Autodesk Fusion 360 part; units mm, degrees
(part 2 of 2)
  spline S375 degree 3 poles (1.9158, -4.1555) (1.6856, -3.9558) (1.3163, -3.6912) (1.1005, -3.5598) knots 0 0 0 0 1 1 1 1
  spline S376 degree 3 poles (1.1005, -3.5598) (0.8754, -3.4317) (0.4108, -3.1073) (0.0566, -2.8267) knots 0 0 0 0 1 1 1 1
  spline S377 degree 3 poles (0.0566, -2.8267) (-0.2941, -2.5554) (-0.6989, -2.2512) (-0.8388, -2.1551) knots 0 0 0 0 1 1 1 1
  spline S378 degree 3 poles (-0.8388, -2.1551) (-0.9788, -2.059) (-1.3388, -1.7911) (-1.6449, -1.556) knots 0 0 0 0 1 1 1 1
  spline S379 degree 3 poles (-1.6449, -1.556) (-1.9417, -1.3175) (-2.3043, -1.0714) (-2.4341, -1.0032) knots 0 0 0 0 1 1 1 1
  spline S380 degree 3 poles (-2.4341, -1.0032) (-2.5639, -0.9349) (-2.7739, -0.7909) (-2.9046, -0.6914) knots 0 0 0 0 1 1 1 1
  spline S381 degree 3 poles (-2.9046, -0.6914) (-3.4695, -0.2355) (-3.9222, -0.4633) (-3.5882, -1.0347) knots 0 0 0 0 1 1 1 1
  spline S382 degree 3 poles (-3.5882, -1.0347) (-3.4574, -1.2496) (-3.4321, -1.3769) (-3.4978, -1.4849) knots 0 0 0 0 1 1 1 1
  spline S383 degree 3 poles (-3.4978, -1.4849) (-3.6891, -1.796) (-4.0336, -2.8979) (-4.0486, -3.2604) knots 0 0 0 0 1 1 1 1
  spline S384 degree 3 poles (-4.0486, -3.2604) (-4.0922, -4.1792) (-3.8414, -5.705) (-3.4803, -6.6971) knots 0 0 0 0 1 1 1 1
  spline S385 degree 3 poles (-3.4803, -6.6971) (-3.1361, -7.6428) (-3.1099, -7.6858) (-2.4943, -8.2808) knots 0 0 0 0 1 1 1 1
  spline S386 degree 3 poles (-2.4943, -8.2808) (-1.8788, -8.8758) (-1.453, -9.1513) (-0.5011, -9.6029) knots 0 0 0 0 1 1 1 1
  spline S387 degree 3 poles (-0.5011, -9.6029) (-0.0425, -9.8244) (1.2112, -10.1242) (1.3873, -10.06) knots 0 0 0 0 1 1 1 1
  spline S388 degree 3 poles (1.3873, -10.06) (1.4337, -10.0432) (1.765, -10.0591) (2.125, -10.0961) knots 0 0 0 0 1 1 1 1
  spline S389 degree 3 poles (2.125, -10.0961) (3.0076, -10.1843) (4.5443, -9.877) (5.7007, -9.3616) knots 0 0 0 0 1 1 1 1
  line L40 (5.7007, -9.3616) -> (6.5613, -8.9854)
  line L41 (6.5613, -8.9854) -> (6.9205, -9.2222)
  spline S390 degree 3 poles (6.9205, -9.2222) (7.1237, -9.3477) (7.3025, -9.4926) (7.3227, -9.5483) knots 0 0 0 0 1 1 1 1
  spline S391 degree 3 poles (7.3227, -9.5483) (7.3396, -9.5946) (7.4922, -9.6966) (7.6659, -9.7699) knots 0 0 0 0 1 1 1 1
  spline S392 degree 3 poles (7.6659, -9.7699) (7.9247, -9.8752) (8.0183, -9.8726) (8.1118, -9.7546) knots 0 0 0 0 1 1 1 1
  spline S393 degree 3 poles (8.1118, -9.7546) (8.2534, -9.5666) (8.2272, -9.2926) (8.0704, -9.2657) knots 0 0 0 0 1 1 1 1
  spline S394 degree 3 poles (5.741, -8.549) (5.6676, -8.6071) (5.0489, -8.8113) (4.3485, -8.9928) knots 0 0 0 0 1 1 1 1
  spline S395 degree 3 poles (4.3485, -8.9928) (3.0596, -9.3464) (2.0565, -9.4175) (0.8476, -9.2695) knots 0 0 0 0 1 1 1 1
  spline S396 degree 3 poles (0.8476, -9.2695) (0.0678, -9.1753) (-1.0477, -8.5628) (-1.8774, -7.7832) knots 0 0 0 0 1 1 1 1
  spline S397 degree 3 poles (-1.8774, -7.7832) (-2.2586, -7.4284) (-2.3859, -7.2228) (-2.7267, -6.4018) knots 0 0 0 0 1 1 1 1
  spline S398 degree 3 poles (-2.7267, -6.4018) (-3.0481, -5.6053) (-3.1283, -5.2985) (-3.1774, -4.6443) knots 0 0 0 0 1 1 1 1
  spline S399 degree 3 poles (-3.1774, -4.6443) (-3.2756, -3.336) (-3.0585, -1.913) (-2.734, -1.7948) knots 0 0 0 0 1 1 1 1
  spline S400 degree 3 poles (-2.734, -1.7948) (-2.6876, -1.778) (-2.5477, -1.874) (-2.4473, -2.0055) knots 0 0 0 0 1 1 1 1
  spline S401 degree 3 poles (-2.4473, -2.0055) (-2.3343, -2.1429) (-2.207, -2.2331) (-2.1606, -2.2162) knots 0 0 0 0 1 1 1 1
  spline S402 degree 3 poles (-2.1606, -2.2162) (-2.1143, -2.1993) (-1.981, -2.2768) (-1.8714, -2.4049) knots 0 0 0 0 1 1 1 1
  spline S403 degree 3 poles (-1.8714, -2.4049) (-1.7559, -2.5204) (-1.5232, -2.6982) (-1.3613, -2.7968) knots 0 0 0 0 1 1 1 1
  spline S404 degree 3 poles (-1.3613, -2.7968) (-1.1868, -2.9012) (-1.0367, -3.0251) (-1.0198, -3.0715) knots 0 0 0 0 1 1 1 1
  spline S405 degree 3 poles (-1.0198, -3.0715) (-0.9995, -3.1271) (-0.841, -3.2164) (-0.6707, -3.2804) knots 0 0 0 0 1 1 1 1
  line L42 (-0.6707, -3.2804) -> (-0.3647, -3.4001)
  line L43 (-0.3647, -3.4001) -> (-0.8376, -3.5722)
  spline S406 degree 3 poles (-0.8376, -3.5722) (-1.3475, -3.7578) (-1.4461, -3.9197) (-1.2437, -4.245) knots 0 0 0 0 1 1 1 1
  spline S407 degree 3 poles (-1.2437, -4.245) (-1.1062, -4.4785) (-0.6307, -4.5154) (0.2358, -4.3575) knots 0 0 0 0 1 1 1 1
  spline S408 degree 3 poles (0.2358, -4.3575) (0.7449, -4.2562) (0.7702, -4.268) (1.6868, -5.0264) knots 0 0 0 0 1 1 1 1
  spline S409 degree 3 poles (1.6868, -5.0264) (1.8976, -5.2017) (2.4237, -5.6087) (2.8698, -5.9399) knots 0 0 0 0 1 1 1 1
  spline S410 degree 3 poles (2.8698, -5.9399) (3.3192, -6.2803) (3.9094, -6.748) (4.1877, -6.9932) knots 0 0 0 0 1 1 1 1
  spline S411 degree 3 poles (4.1877, -6.9932) (4.466, -7.2385) (4.7788, -7.4921) (4.896, -7.5545) knots 0 0 0 0 1 1 1 1
  spline S412 degree 3 poles (4.896, -7.5545) (5.197, -7.7179) (5.7526, -8.1772) (5.8159, -8.3222) knots 0 0 0 0 1 1 1 1
  spline S413 degree 3 poles (5.8159, -8.3222) (5.8488, -8.3837) (5.8109, -8.4815) (5.741, -8.549) knots 0 0 0 0 1 1 1 1
  spline S414 degree 3 poles (-3.274, 16.9406) (-3.4561, 17.0948) (-3.6786, 17.0138) (-4.2602, 16.5921) knots 0 0 0 0 1 1 1 1
  spline S415 degree 3 poles (-4.2602, 16.5921) (-4.6917, 16.2775) (-4.7473, 16.2573) (-5.5009, 16.193) knots 0 0 0 0 1 1 1 1
  spline S416 degree 3 poles (-5.5009, 16.193) (-6.7435, 16.0873) (-8.9021, 15.2386) (-10.4235, 14.2543) knots 0 0 0 0 1 1 1 1
  spline S417 degree 3 poles (-10.4235, 14.2543) (-10.8128, 13.9971) (-11.605, 13.2888) (-12.2025, 12.6513) knots 0 0 0 0 1 1 1 1
  spline S418 degree 3 poles (-12.2025, 12.6513) (-13.352, 11.4244) (-15.0798, 7.4879) (-15.2033, 5.8365) knots 0 0 0 0 1 1 1 1
  spline S419 degree 3 poles (-15.2033, 5.8365) (-15.2159, 5.6114) (-15.2756, 5.2851) (-15.3236, 5.0997) knots 0 0 0 0 1 1 1 1
  spline S420 degree 3 poles (-15.3236, 5.0997) (-15.4323, 4.7346) (-15.4883, 3.1287) (-15.4347, 1.5102) knots 0 0 0 0 1 1 1 1
  spline S421 degree 3 poles (-15.4347, 1.5102) (-15.3878, -0.3208) (-14.9842, -2.295) (-14.2595, -4.2573) knots 0 0 0 0 1 1 1 1
  spline S422 degree 3 poles (-14.2595, -4.2573) (-13.8174, -5.4719) (-13.6622, -5.7829) (-13.0601, -6.6873) knots 0 0 0 0 1 1 1 1
  spline S423 degree 3 poles (-13.0601, -6.6873) (-12.5718, -7.4231) (-12.2201, -7.8411) (-11.8592, -8.1402) knots 0 0 0 0 1 1 1 1
  spline S424 degree 3 poles (-11.8592, -8.1402) (-11.5692, -8.3602) (-11.1374, -8.7385) (-10.8971, -8.9661) knots 0 0 0 0 1 1 1 1
  spline S425 degree 3 poles (-10.8971, -8.9661) (-10.4359, -9.3967) (-9.5489, -9.9874) (-8.7513, -10.3901) knots 0 0 0 0 1 1 1 1
  spline S426 degree 3 poles (-8.7513, -10.3901) (-7.9537, -10.7928) (-4.9869, -11.6451) (-4.718, -11.5472) knots 0 0 0 0 1 1 1 1
  spline S427 degree 3 poles (-4.718, -11.5472) (-4.4121, -11.4358) (-3.9341, -11.5664) (-2.8785, -12.0432) knots 0 0 0 0 1 1 1 1
  spline S428 degree 3 poles (-2.8785, -12.0432) (-1.7057, -12.5824) (-1.3795, -12.6421) (-1.3324, -12.31) knots 0 0 0 0 1 1 1 1
  spline S429 degree 3 poles (-1.3324, -12.31) (-1.3054, -12.1531) (-1.4429, -12.0352) (-2.0415, -11.7175) knots 0 0 0 0 1 1 1 1
  spline S430 degree 3 poles (-2.0415, -11.7175) (-2.447, -11.4976) (-2.8113, -11.3047) (-2.8585, -11.2904) knots 0 0 0 0 1 1 1 1
  spline S431 degree 3 poles (-2.8585, -11.2904) (-3.2075, -11.1969) (-4.9717, -9.1194) (-5.6253, -8.0448) knots 0 0 0 0 1 1 1 1
  spline S432 degree 3 poles (-5.6253, -8.0448) (-6.3675, -6.8134) (-6.6982, -6.0203) (-7.1606, -4.4035) knots 0 0 0 0 1 1 1 1
  spline S433 degree 3 poles (-7.1606, -4.4035) (-7.807, -2.1083) (-8.1042, -0.7149) (-8.1424, 0.2267) knots 0 0 0 0 1 1 1 1
  spline S434 degree 3 poles (-8.1424, 0.2267) (-8.1712, 0.7098) (-8.2212, 1.5106) (-8.266, 2.0088) knots 0 0 0 0 1 1 1 1
  spline S435 degree 3 poles (-8.266, 2.0088) (-8.4807, 4.1567) (-8.2895, 7.5549) (-7.8887, 8.8768) knots 0 0 0 0 1 1 1 1
  spline S436 degree 3 poles (-7.8887, 8.8768) (-7.7851, 9.198) (-7.6731, 9.6693) (-7.6361, 9.9137) knots 0 0 0 0 1 1 1 1
  spline S437 degree 3 poles (-7.6361, 9.9137) (-7.5376, 10.5376) (-7.3708, 10.9448) (-6.8249, 11.9835) knots 0 0 0 0 1 1 1 1
  spline S438 degree 3 poles (-6.8249, 11.9835) (-6.5637, 12.4776) (-6.2343, 13.1015) (-6.0919, 13.3739) knots 0 0 0 0 1 1 1 1
  spline S439 degree 3 poles (-6.0919, 13.3739) (-5.9529, 13.6555) (-5.8063, 13.8873) (-5.7784, 13.8974) knots 0 0 0 0 1 1 1 1
  spline S440 degree 3 poles (-5.7784, 13.8974) (-5.7414, 13.9109) (-5.545, 14.1504) (-5.3343, 14.4371) knots 0 0 0 0 1 1 1 1
  spline S441 degree 3 poles (-5.3343, 14.4371) (-4.8709, 15.0678) (-4.0425, 15.9363) (-3.5713, 16.2863) knots 0 0 0 0 1 1 1 1
  spline S442 degree 3 poles (-3.5713, 16.2863) (-3.1491, 16.5975) (-3.0724, 16.7619) (-3.274, 16.9406) knots 0 0 0 0 1 1 1 1
  spline S443 degree 3 poles (-6.1294, 14.8617) (-6.4572, 14.5219) (-7.5618, 12.5658) (-7.6477, 12.1671) knots 0 0 0 0 1 1 1 1
  spline S444 degree 3 poles (-7.6477, 12.1671) (-7.7504, 11.6992) (-7.7007, 11.7068) (-9.8958, 11.6218) knots 0 0 0 0 1 1 1 1
  spline S445 degree 3 poles (-9.8958, 11.6218) (-10.2574, 11.6057) (-10.8981, 11.5195) (-12.085, 11.3186) knots 0 0 0 0 1 1 1 1
  spline S446 degree 3 poles (-12.085, 11.3186) (-12.2713, 11.2822) (-12.1381, 11.4357) (-10.5706, 13.0143) knots 0 0 0 0 1 1 1 1
  spline S447 degree 3 poles (-10.5706, 13.0143) (-10.1181, 13.473) (-8.5225, 14.3687) (-7.0997, 14.9601) knots 0 0 0 0 1 1 1 1
  spline S448 degree 3 poles (-7.0997, 14.9601) (-5.8312, 15.4848) (-5.3254, 15.5954) (-5.7005, 15.2699) knots 0 0 0 0 1 1 1 1
  spline S449 degree 3 poles (-5.7005, 15.2699) (-5.8134, 15.1763) (-5.9988, 14.9933) (-6.1294, 14.8617) knots 0 0 0 0 1 1 1 1
  spline S450 degree 3 poles (-8.2095, 10.6815) (-8.2491, 10.6461) (-8.3553, 10.303) (-8.4538, 9.9101) knots 0 0 0 0 1 1 1 1
  spline S451 degree 3 poles (-8.4538, 9.9101) (-8.5523, 9.5173) (-8.6643, 9.1615) (-8.7064, 9.1042) knots 0 0 0 0 1 1 1 1
  spline S452 degree 3 poles (-8.7064, 9.1042) (-8.8151, 8.9701) (-9.0078, 7.7974) (-9.0085, 7.2512) knots 0 0 0 0 1 1 1 1
  spline S453 degree 3 poles (-9.0085, 7.2512) (-9.0193, 6.5017) (-9.1398, 6.3424) (-9.7307, 6.2638) knots 0 0 0 0 1 1 1 1
  spline S454 degree 3 poles (-9.7307, 6.2638) (-10.0013, 6.2283) (-10.3005, 6.2139) (-10.3882, 6.224) knots 0 0 0 0 1 1 1 1
  spline S455 degree 3 poles (-10.3882, 6.224) (-10.7642, 6.2761) (-12.8463, 6.0538) (-13.8494, 5.8672) knots 0 0 0 0 1 1 1 1
  spline S456 degree 3 poles (-13.8494, 5.8672) (-14.3181, 5.7701) (-14.4142, 5.8612) (-14.2879, 6.2641) knots 0 0 0 0 1 1 1 1
  spline S457 degree 3 poles (-14.2879, 6.2641) (-13.8635, 7.6367) (-13.6756, 8.188) (-13.5156, 8.6138) knots 0 0 0 0 1 1 1 1
  spline S458 degree 3 poles (-13.5156, 8.6138) (-13.4137, 8.8819) (-13.3362, 9.1306) (-13.3497, 9.1677) knots 0 0 0 0 1 1 1 1
  spline S459 degree 3 poles (-13.3497, 9.1677) (-13.3598, 9.1955) (-13.2208, 9.4771) (-13.0354, 9.7756) knots 0 0 0 0 1 1 1 1
  spline S460 degree 3 poles (-13.0354, 9.7756) (-12.7456, 10.2486) (-12.6267, 10.3548) (-12.2651, 10.4865) knots 0 0 0 0 1 1 1 1
  spline S461 degree 3 poles (-12.2651, 10.4865) (-11.8108, 10.6518) (-11.2696, 10.7228) (-10.6542, 10.7053) knots 0 0 0 0 1 1 1 1
  spline S462 degree 3 poles (-10.6542, 10.7053) (-10.4544, 10.7045) (-9.8155, 10.7376) (-9.2397, 10.8001) knots 0 0 0 0 1 1 1 1
  spline S463 degree 3 poles (-9.2397, 10.8001) (-8.3023, 10.8788) (-8.03, 10.8519) (-8.2095, 10.6815) knots 0 0 0 0 1 1 1 1
  spline S464 degree 3 poles (-9.1436, 4.997) (-9.2344, 4.3234) (-9.0243, 0.6303) (-8.8292, -0.5692) knots 0 0 0 0 1 1 1 1
  spline S465 degree 3 poles (-8.8292, -0.5692) (-8.7017, -1.3523) (-8.7118, -1.44) (-8.9014, -1.4671) knots 0 0 0 0 1 1 1 1
  spline S466 degree 3 poles (-8.9014, -1.4671) (-9.0102, -1.4856) (-9.4325, -1.5658) (-9.8329, -1.6486) knots 0 0 0 0 1 1 1 1
  spline S467 degree 3 poles (-9.8329, -1.6486) (-10.2333, -1.7313) (-10.9734, -1.8327) (-11.4809, -1.8809) knots 0 0 0 0 1 1 1 1
  spline S468 degree 3 poles (-11.4809, -1.8809) (-11.9791, -1.9257) (-12.7099, -2.0237) (-13.101, -2.1031) knots 0 0 0 0 1 1 1 1
  spline S469 degree 3 poles (-13.101, -2.1031) (-13.4829, -2.1791) (-13.8909, -2.212) (-14.0106, -2.1716) knots 0 0 0 0 1 1 1 1
  spline S470 degree 3 poles (-14.0106, -2.1716) (-14.2087, -2.1177) (-14.2222, -2.0806) (-14.2899, -1.3177) knots 0 0 0 0 1 1 1 1
  spline S471 degree 3 poles (-14.2899, -1.3177) (-14.3271, -0.8693) (-14.4015, -0.3188) (-14.4487, -0.0735) knots 0 0 0 0 1 1 1 1
  spline S472 degree 3 poles (-14.4487, -0.0735) (-14.6438, 0.895) (-14.7224, 4.573) (-14.5581, 4.9583) knots 0 0 0 0 1 1 1 1
  spline S473 degree 3 poles (-14.5581, 4.9583) (-14.511, 5.0594) (-12.1186, 5.3527) (-10.4858, 5.4535) knots 0 0 0 0 1 1 1 1
  spline S474 degree 3 poles (-10.4858, 5.4535) (-9.9311, 5.4873) (-9.4143, 5.5389) (-9.3494, 5.5625) knots 0 0 0 0 1 1 1 1
  spline S475 degree 3 poles (-9.3494, 5.5625) (-9.1825, 5.6233) (-9.0881, 5.3637) (-9.1436, 4.997) knots 0 0 0 0 1 1 1 1
  spline S476 degree 3 poles (-4.8203, -10.7759) (-5.1811, -10.7077) (-7.1202, -10.1114) (-8.0872, -9.7914) knots 0 0 0 0 1 1 1 1
  spline S477 degree 3 poles (-8.0872, -9.7914) (-8.292, -9.719) (-8.7321, -9.4906) (-9.0534, -9.2715) knots 0 0 0 0 1 1 1 1
  spline S478 degree 3 poles (-9.0534, -9.2715) (-9.3839, -9.0558) (-9.8282, -8.7871) (-10.0432, -8.6868) knots 0 0 0 0 1 1 1 1
  spline S479 degree 3 poles (-10.0432, -8.6868) (-10.2523, -8.5739) (-10.3957, -8.4686) (-10.34, -8.4483) knots 0 0 0 0 1 1 1 1
  spline S480 degree 3 poles (-10.34, -8.4483) (-10.2937, -8.4314) (-9.7213, -8.3596) (-9.0646, -8.2886) knots 0 0 0 0 1 1 1 1
  spline S481 degree 3 poles (-9.0646, -8.2886) (-8.4046, -8.2269) (-7.6274, -8.112) (-7.3357, -8.0479) knots 0 0 0 0 1 1 1 1
  spline S482 degree 3 poles (-7.3357, -8.0479) (-7.0474, -7.9744) (-6.7861, -7.9423) (-6.7448, -7.9693) knots 0 0 0 0 1 1 1 1
  spline S483 degree 3 poles (-6.7448, -7.9693) (-6.7128, -7.9996) (-6.4488, -8.4076) (-6.1612, -8.8804) knots 0 0 0 0 1 1 1 1
  spline S484 degree 3 poles (-6.1612, -8.8804) (-5.8281, -9.4206) (-5.4401, -9.9095) (-5.0978, -10.2154) knots 0 0 0 0 1 1 1 1
  spline S485 degree 3 poles (-5.0978, -10.2154) (-4.435, -10.8247) (-4.4089, -10.8677) (-4.8203, -10.7759) knots 0 0 0 0 1 1 1 1
  spline S486 degree 3 poles (-7.8137, -5.0613) (-7.602, -5.7297) (-7.3666, -6.3475) (-7.2106, -6.5743) knots 0 0 0 0 1 1 1 1
  spline S487 degree 3 poles (-7.2106, -6.5743) (-7.0798, -6.7892) (-6.9837, -6.9957) (-7.0073, -7.0463) knots 0 0 0 0 1 1 1 1
  spline S488 degree 3 poles (-7.0073, -7.0463) (-7.0873, -7.2014) (-9.204, -7.5308) (-10.5317, -7.6045) knots 0 0 0 0 1 1 1 1
  spline S489 degree 3 poles (-10.5317, -7.6045) (-10.943, -7.6283) (-11.1133, -7.5642) (-11.4574, -7.3115) knots 0 0 0 0 1 1 1 1
  spline S490 degree 3 poles (-11.4574, -7.3115) (-11.6808, -7.1303) (-11.9675, -6.8041) (-12.0831, -6.5732) knots 0 0 0 0 1 1 1 1
  spline S491 degree 3 poles (-12.0831, -6.5732) (-12.2045, -6.3549) (-12.4525, -5.9621) (-12.6279, -5.7109) knots 0 0 0 0 1 1 1 1
  spline S492 degree 3 poles (-12.6279, -5.7109) (-12.8126, -5.4632) (-13.1593, -4.7703) (-13.4098, -4.1685) knots 0 0 0 0 1 1 1 1
  line L44 (-13.4098, -4.1685) -> (-13.8544, -3.0913)
  line L45 (-13.8544, -3.0913) -> (-13.3832, -2.9723)
  spline S493 degree 3 poles (-13.3832, -2.9723) (-12.8564, -2.833) (-11.7521, -2.6936) (-11.296, -2.7061) knots 0 0 0 0 1 1 1 1
  spline S494 degree 3 poles (-11.296, -2.7061) (-11.1401, -2.7019) (-10.5711, -2.6208) (-10.0526, -2.5161) knots 0 0 0 0 1 1 1 1
  spline S495 degree 3 poles (-10.0526, -2.5161) (-8.4848, -2.2079) (-8.677, -2.1414) (-8.4011, -3.1015) knots 0 0 0 0 1 1 1 1
  spline S496 degree 3 poles (-8.4011, -3.1015) (-8.2669, -3.5567) (-8.0087, -4.4392) (-7.8137, -5.0613) knots 0 0 0 0 1 1 1 1
  spline S497 degree 3 poles (-23.8057, -15.418) (-24.9076, -14.8425) (-24.9237, -14.8273) (-24.8512, -14.6225) knots 0 0 0 0 1 1 1 1
  spline S498 degree 3 poles (-24.8512, -14.6225) (-24.8133, -14.5247) (-24.6979, -14.4092) (-24.5866, -14.3687) knots 0 0 0 0 1 1 1 1
  spline S499 degree 3 poles (-24.5866, -14.3687) (-24.3118, -14.2581) (-24.0944, -13.8745) (-24.1316, -13.5415) knots 0 0 0 0 1 1 1 1
  spline S500 degree 3 poles (-24.1316, -13.5415) (-24.217, -12.8166) (-27.0774, -12.1987) (-28.2794, -12.6467) knots 0 0 0 0 1 1 1 1
  spline S501 degree 3 poles (-28.2794, -12.6467) (-28.6596, -12.785) (-28.8189, -12.8955) (-28.9073, -13.0852) knots 0 0 0 0 1 1 1 1
  spline S502 degree 3 poles (-28.9073, -13.0852) (-29.0666, -13.4267) (-28.9274, -13.4915) (-28.3349, -13.3599) knots 0 0 0 0 1 1 1 1
  spline S503 degree 3 poles (-28.3349, -13.3599) (-27.5282, -13.1817) (-26.5385, -13.189) (-25.7536, -13.3549) knots 0 0 0 0 1 1 1 1
  spline S504 degree 3 poles (-25.7536, -13.3549) (-25.3641, -13.4441) (-25.0303, -13.5536) (-25.0134, -13.6) knots 0 0 0 0 1 1 1 1
  spline S505 degree 3 poles (-25.0134, -13.6) (-24.9999, -13.6371) (-25.117, -13.8057) (-25.2687, -13.9659) knots 0 0 0 0 1 1 1 1
  spline S506 degree 3 poles (-25.2687, -13.9659) (-25.433, -14.1202) (-25.5721, -14.2863) (-25.5898, -14.3243) knots 0 0 0 0 1 1 1 1
  spline S507 degree 3 poles (-25.5898, -14.3243) (-25.6075, -14.3622) (-25.6917, -14.4769) (-25.7794, -14.5823) knots 0 0 0 0 1 1 1 1
  spline S508 degree 3 poles (-25.7794, -14.5823) (-25.8797, -14.6818) (-25.9285, -14.8361) (-25.8948, -14.9288) knots 0 0 0 0 1 1 1 1
  spline S509 degree 3 poles (-25.8948, -14.9288) (-25.8644, -15.0122) (-25.4007, -15.3055) (-24.8754, -15.5658) knots 0 0 0 0 1 1 1 1
  spline S510 degree 3 poles (-24.8754, -15.5658) (-24.356, -15.8388) (-23.9277, -16.0924) (-23.942, -16.1396) knots 0 0 0 0 1 1 1 1
  spline S511 degree 3 poles (-23.942, -16.1396) (-23.9471, -16.1834) (-24.1831, -16.3428) (-24.4696, -16.4786) knots 0 0 0 0 1 1 1 1
  spline S512 degree 3 poles (-24.4696, -16.4786) (-25.2948, -16.8945) (-25.5232, -17.1036) (-25.4287, -17.3632) knots 0 0 0 0 1 1 1 1
  spline S513 degree 3 poles (-25.4287, -17.3632) (-25.3308, -17.6321) (-25.0964, -17.8723) (-24.7356, -18.056) knots 0 0 0 0 1 1 1 1
  spline S514 degree 3 poles (-24.7356, -18.056) (-24.3806, -18.2523) (-24.5214, -18.356) (-25.0718, -18.3149) knots 0 0 0 0 1 1 1 1
  spline S515 degree 3 poles (-25.0718, -18.3149) (-25.5566, -18.2813) (-25.9536, -18.3733) (-25.9898, -18.5335) knots 0 0 0 0 1 1 1 1
  spline S516 degree 3 poles (-25.9898, -18.5335) (-26.0007, -18.59) (-25.8877, -18.7273) (-25.741, -18.8419) knots 0 0 0 0 1 1 1 1
  spline S517 degree 3 poles (-25.741, -18.8419) (-25.3995, -19.1166) (-24.3062, -19.1492) (-23.9134, -18.9012) knots 0 0 0 0 1 1 1 1
  spline S518 degree 3 poles (-23.9134, -18.9012) (-23.5055, -18.6373) (-23.5401, -18.3979) (-24.0553, -17.8189) knots 0 0 0 0 1 1 1 1
  spline S519 degree 3 poles (-24.0553, -17.8189) (-24.3033, -17.5416) (-24.5132, -17.282) (-24.5234, -17.2542) knots 0 0 0 0 1 1 1 1
  spline S520 degree 3 poles (-24.5234, -17.2542) (-24.5369, -17.2171) (-24.2966, -17.0982) (-23.9814, -16.9835) knots 0 0 0 0 1 1 1 1
  spline S521 degree 3 poles (-23.9814, -16.9835) (-23.4807, -16.8012) (-23.3981, -16.7397) (-23.2448, -16.4108) knots 0 0 0 0 1 1 1 1
  spline S522 degree 3 poles (-23.2448, -16.4108) (-23.1504, -16.2085) (-23.1008, -15.9699) (-23.1311, -15.8865) knots 0 0 0 0 1 1 1 1
  spline S523 degree 3 poles (-23.1311, -15.8865) (-23.1615, -15.803) (-23.4608, -15.5865) (-23.8057, -15.418) knots 0 0 0 0 1 1 1 1
  dimension "d4" = 35
  dimension "d5" = 35
  constraint coincident A0.centre L0.start
  constraint horizontal L0
  constraint perpendicular L0 L1
  measures "d4" distance of A0.centre L0.end
  measures "d5" distance of L0.end L1.end
extrude "Extrude2" cut sketch "Sketch2" against normal blind 1 contours S160 S161 S162 S163 S164 S165 S166 S167 S168 S169 L18 L19 S170 S171 S172 S173 S174 S175 S176 S177 S178 S179 S180 S181 S182 S183 S184 L20 L21 S185 S186 S187 S188 S189 S190 S191 S192 S193 S194 S195 S196 S197 S198 S199 S200 S201 S202 S203 S204 S205 S206 S207 S208 S209 S210 S211 S212 S213 S214 S215 S216 S217 S218 L22 L23 S219 L24 L25 S220 S221 S222 S223 S224 S225 S226 S227 S228 S229 S230 S231 S232 S233 S234 S235 S236 S237 S238 L26 L27 S239 S240 S241 S242 S243 S244 S245 S246 S247 S248 S249 S250 L28 L29 S251 S252 S253 S254 S255 S256 S257 S258 S259 S260 S261 S262 S263 S264 S265 S266 S267 S268 S269 S270 S271 S272 S273 S274 S275 S276 S277 S278 S279 S280 S281 L30 L31 S282 S283 S284 S285 S286 S287 S288 S289 S290 S291 S292 S293 S294 S295 S296 S297 S298 S299 S300 S301 S302 S303 S304 S305 S306 S307 S308 L32 L33 S309 S310 S311 L34 L35 S312 S313 S314 S315 S316 S317 S318 S319 S320 S321 S322 S323 S324 S325 S326 S327 S328 L36 L37 S329 S330 S331 S332 S333 S334 | S335 S336 S337 S338 S339 S340 S341 S342 | S357 S358 S359 S360 S361 S362 S363 S364 S365 S366 S367 S368 S369 | S394 S395 S396 S397 S398 S399 S400 S401 S402 S403 S404 S405 L42 L43 S406 S407 S408 S409 S410 S411 S412 S413 | S443 S444 S445 S446 S447 S448 S449 | S450 S451 S452 S453 S454 S455 S456 S457 S458 S459 S460 S461 S462 S463 | S464 S465 S466 S467 S468 S469 S470 S471 S472 S473 S474 S475 | S476 S477 S478 S479 S480 S481 S482 S483 S484 S485 | S486 S487 S488 S489 S490 S491 S492 L44 L45 S493 S494 S495 S496
extrude "Extrude3" add 1 faces at (-11.2989, -20.8875, 0) along direction (0, 0, -1) blind 1
